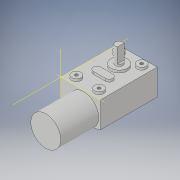
# Autodesk Inventor part: BT001_trajan20_21
Saved by Autodesk Inventor 2022.2 (Build 262287000, 287)
## iProperties
Company: HTBLA Kaindorf
RuleStatus: InUse
Created: 2022-06-05
Part Number: BT001_trajan20_21
Project: Getriebemotor
Material: Generisch
Description: Masterskizze
Document SubType Name: Modeling
Designer: trajan20
Density: 1 g/cm^3
Appearance: Vorgabe
Mass: 47.3308 g
Surface Area: 93.2862 cm^2
Volume: 47.3308 cm^3
AfterDocNew0: iProperties-Editor_aufrufen
Author: jan
Keywords: 2021
Autodesk Inventor part; units mm, degrees
ref_plane "YZ Plane" through (0, 0, 0) normal (1, 0, 0) x (0, 1, 0)
ref_plane "XZ Plane" through (0, 0, 0) normal (0, 1, 0) x (-1, 0, 0)
ref_plane "XY Plane" through (0, 0, 0) normal (0, 0, 1) x (1, 0, 0)
sketch "Skizze3" plane through (0, 0, 0) normal (0, 0, 1) x (1, 0, 0)
  line L0 (0, 0) -> (-45.87, 0)
  line L1 (-45.87, 0) -> (-45.87, 31.87)
  line L2 (-45.87, 31.87) -> (0, 31.87)
  line L3 (0, 31.87) -> (0, 0)
  circle A0 centre (-40.12, 25.12) radius 3.75
  line L4 (-6.8112, 15.935) -> (-34.2962, 15.935) construction
  circle A1 centre (-31.07, 15.935) radius 6.65
  circle A2 centre (-31.07, 15.935) radius 3
  circle A3 centre (-40.12, 6.75) radius 3.75
  circle A4 centre (-5.75, 25.12) radius 3.75
  circle A5 centre (-5.75, 6.75) radius 3.75
  line L5 (-18.15, 11) -> (-18.15, 20.87) construction
  line L6 (-15.15, 11) -> (-15.15, 20.87)
  line L7 (-21.15, 20.87) -> (-21.15, 11)
  arc A6 (-21.15, 11) -> (-15.15, 11) centre (-18.15, 11) ccw
  arc A7 (-15.15, 20.87) -> (-21.15, 20.87) centre (-18.15, 20.87) ccw
  point P0 (0, 15.935)
  point P1 (-18.15, 15.935)
  point P2 (-18.15, 23.87)
  point P3 (-18.15, 8)
  dimension "d5" = 6.75
  dimension "d6" = 5.75
  dimension "d7" = 7.5
  dimension "d9" = 45.87
  dimension "d10" = 31.87
  dimension "d11" = 14.8
  dimension "d12" = 13.3
  dimension "d13" = 6
  dimension "d14" = 6.75
  dimension "d15" = 6.75
  dimension "d16" = 6.75
  dimension "d17" = 5.75
  dimension "d18" = 5.75
  dimension "d19" = 5.75
  dimension "d20" = 7.5
  dimension "d21" = 7.5
  dimension "d22" = 7.5
  dimension "d23" = 15.87
  dimension "d24" = 18.15
  dimension "d25" = 6
  constraints: 18 end point, 8 centre point, 6 coincident, 6 point on circle, 4 tangent, 3 parallel, 3 point on line, 2 horizontal, 2 midpoint, 2 perpendicular
  measures "d5" distance from line of L2 point (-40.12, 25.12)
  measures "d6" distance from line of L1 point (-40.12, 25.12)
  measures "d7" diameter of A0
  measures "d9" distance of L1.end L2.end
  measures "d10" distance between parallel lines of L0 L2
  measures "d11" distance from line of L1 point (-31.07, 15.935)
  measures "d12" diameter of A1
  measures "d13" diameter of A2
  measures "d14" distance from line of L2 point (-5.75, 25.12)
  measures "d15" distance from line of L0 point (-5.75, 6.75)
  measures "d16" distance from line of L0 point (-40.12, 6.75)
  measures "d17" distance from line of L1 point (-40.12, 6.75)
  measures "d18" distance from line of L3 point (-5.75, 6.75)
  measures "d19" distance from line of point (-5.75, 25.12) L3
  measures "d20" diameter of A3
  measures "d21" diameter of A5
  measures "d22" diameter of A4
  measures "d23" distance of point (-18.15, 23.87) point (-18.15, 8)
  measures "d24" distance between parallel lines of L3 L5
  measures "d25" distance between parallel lines of L7 L6
extrude "Extrusion3" add sketch "Skizze3" against normal blind 22.25 contours L0 L1 L2 L3 | A0 | A1 | A2 | A3 | A4 | A5 | A6 L7 A7 L6
extrude "Extrusion4" add sketch "Skizze3" along normal blind 2 contours A0 | A1 | A3 | A4 | A5 | A6 L7 A7 L6
extrude "Extrusion5" add sketch "Skizze3" along normal blind 15.5 contours A2
sketch "Skizze4" plane through (0, 0, 0) normal (1, 0, 0) x (0, 0, -1)
  line L0 (0, 31.87) -> (22.25, 31.87) projected
  line L1 (0, 0) -> (0, 31.87) projected
  circle A0 centre (13.075, 18.495) radius 12.075
  dimension "d33" = 13.375
  dimension "d34" = 13.075
  dimension "d35" = 24.15
  constraints: 1 centre point, 1 coincident
  measures "d33" distance from line of L0 point (13.075, 18.495)
  measures "d34" distance from line of L1 point (13.075, 18.495)
  measures "d35" diameter of A0
extrude "Extrusion6" add sketch "Skizze4" along normal blind 30.75
sketch "Skizze5" plane through (-5.75, 25.12, 2) normal (0, 0, 1) x (1, 0, 0)
  circle A0 centre (-34.37, 0) radius 3.75 projected
  circle A1 centre (-34.37, -18.37) radius 3.75 projected
  circle A2 centre (0, -18.37) radius 3.75 projected
  circle A3 centre (0, 0) radius 3.75 projected
  circle A4 centre (0, -18.37) radius 3.75 projected
  point P0 (5.75, -25.12)
  constraints: 4 coincident
hole "Bohrung1" at (-5.75, 25.12, 2) at (-5.75, 6.75, 2) at (-40.12, 6.75, 2) at (-40.12, 25.12, 2) direction (0, 0, -1) diameter 2.013 depth 4.15 tip angle 118 thread size "M2.5x0.45" class "6H" standard "ISO Metric profile"
ref_plane "Arbeitsebene1" through (-28.07, 15.935, 0) normal (-1, 0, 0) x (0, 0, 1)
sketch "Skizze6" plane through (-28.07, 15.935, 0) normal (-1, 0, 0) x (0, 0, 1)
  line L0 (15.5, -3) -> (15.5, 3) projected
  line L1 (2, 3) -> (15.5, 3) projected
  line L2 (15.5, 3) -> (3.5, 3)
  line L3 (3.5, 3) -> (3.5, 1.25)
  line L4 (3.5, 1.25) -> (15.5, 1.25)
  line L5 (15.5, 1.25) -> (15.5, 3)
  point P0 (0, -15.935)
  point P1 (3.5, 3)
  point P2 (3.5, 2.125)
  dimension "d49" = 12
  dimension "d50" = 1.75
  constraints: 8 end point, 2 parallel, 1 horizontal, 1 midpoint, 1 perpendicular
  measures "d49" distance from line of L5 point (3.5, 2.125)
  measures "d50" distance between parallel lines of L4 L1
extrude "Extrusion7" cut sketch "Skizze6" along normal blind 30.75 and the other way blind 15.375
chamfer "Fase1" distance 0.25 angle 45 4 edges at (-40.12, 26.1265, 2) (-40.12, 7.7565, 2) (-5.75, 7.7565, 2) (-5.75, 26.1265, 2)
chamfer "Fase2" distance 4.5 distance2 1.25 3 edges at (-22.935, 31.87, -22.25) (-45.87, 15.935, -22.25) (-22.935, 0, -22.25) measured on face at (-22.935, 31.37, -22.25) measured on face at (-45.37, 15.935, -22.25) measured on face at (-22.935, 0.5, -22.25)
equation "\"d5\" = schraube_p_x"
equation "\"d6\" = schraube_p_y"
equation "\"d7\" = schraube_d"
equation "\"d9\" = gh_l"
equation "\"d10\" = gh_b"
equation "\"d11\" = s_p_y"
equation "\"d12\" = s_d_u"
equation "\"d13\" = s_d"
equation "\"d14\" = d5"
equation "\"d15\" = d5"
equation "\"d16\" = d5"
equation "\"d17\" = d6"
equation "\"d18\" = d6"
equation "\"d19\" = d6"
equation "\"d20\" = d7"
equation "\"d21\" = d7"
equation "\"d22\" = d7"
equation "\"d23\" = nut_l"
equation "\"d24\" = nut_p_x_neg"
equation "\"d25\" = nut_b"
equation "\"d26\" = gh_h"
equation "\"d28\" = Absatz_h"
equation "\"d30\" = s_h"
equation "\"d33\" = m_p_xn"
equation "\"d34\" = m_p_z_neg"
equation "\"d35\" = M_d"
equation "\"d36\" = M_l"
equation "\"d45\" = M_l"
equation "\"s_h\" = 15.5"
equation "\"schraube_p_x\" = 6.75"
equation "\"s_p_y\" = 14.8"
equation "\"Absatz_h\" = 2"
equation "\"schraube_d\" = 7.5"
equation "\"gh_h\" = 22.25"
equation "\"M_d\" = 24.15"
equation "\"s_d\" = 6"
equation "\"M_l\" = 30.75"
equation "\"schraube_p_y\" = 5.75"
equation "\"s_d_u\" = 13.3"
equation "\"gs_h\" = 37.75"
equation "\"gh_l\" = 45.87"
equation "\"gh_b\" = 31.87"
equation "\"nut_p_x_neg\" = 18.15"
equation "\"nut_l\" = 15.87"
equation "\"nut_b\" = 6"
equation "\"m_p_z_neg\" = 13.075"
equation "\"m_p_xn\" = 13.375"
